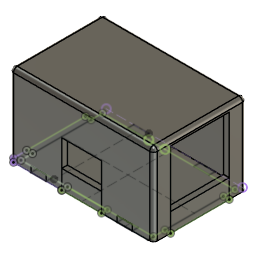
Thermux Temperature Node (Autodesk Fusion 360 design; units mm, degrees)
Autodesk Fusion 360 part; units mm, degrees
note: some values were not read from the file. Chosen so that the rebuilt part matches the saved one: which face or edge a step refers to.
sketch "Sketch1" plane through (0, 0, 0) normal (0, 0, 1) x (1, 0, 0) in component "Lid"
  line L0 (-19, 12.25) -> (19, 12.25)
  line L1 (19, 12.25) -> (19, -12.25)
  line L2 (19, -12.25) -> (-19, -12.25)
  line L3 (-19, -12.25) -> (-19, 12.25)
  line L4 (-19, 12.25) -> (19, -12.25) construction
  line L5 (19, 12.25) -> (-19, -12.25) construction
  line L6 (-17.5, 10.75) -> (17.5, 10.75)
  line L7 (17.5, 10.75) -> (17.5, -10.75)
  line L8 (17.5, -10.75) -> (-17.5, -10.75)
  line L9 (-17.5, -10.75) -> (-17.5, 10.75)
  line L10 (-5.25, -10.75) -> (5.25, -10.75)
  line L11 (5.25, -10.75) -> (5.25, -12.25)
  line L12 (5.25, -12.25) -> (-5.25, -12.25)
  line L13 (-5.25, -12.25) -> (-5.25, -10.75)
  line L14 (0, 12.25) -> (0, -12.25) construction
  line L15 (-19, 0) -> (19, 0) construction
  line L16 (-19, 7.75) -> (-17.5, 7.75)
  line L17 (-17.5, 7.75) -> (-17.5, -7.75)
  line L18 (-17.5, -7.75) -> (-19, -7.75)
  line L19 (-19, -7.75) -> (-19, 7.75)
  line L20 (17.5, 7.75) -> (19, 7.75)
  line L21 (19, 7.75) -> (19, -7.75)
  line L22 (19, -7.75) -> (17.5, -7.75)
  line L23 (17.5, -7.75) -> (17.5, 7.75)
  circle A0 centre (-3.125, 8.125) radius 1.125
  circle A1 centre (-3.125, 8.125) radius 2.125
  line L24 (-4.25, 12.25) -> (-4.25, -12.25) construction
  line L25 (-17.5, 9.25) -> (17.5, 9.25) construction
  line L26 (-5.25, 8.125) -> (-5.25, 10.75)
  line L27 (-1, 8.125) -> (-1, 10.75)
  dimension "d3" = 1.5
  dimension "d4" = 10.5
  dimension "d7" = 15.5
  dimension "d8" = 15.5
  dimension "d9" = 2.25
  dimension "d10" = 1
  dimension "d11" = 13.25
  dimension "d12" = 1.5
  dimension "d34" = 35
  dimension "d35" = 21.5
  constraint horizontal L0
  constraint perpendicular L0 L1
  constraint parallel L0 L2
  constraint parallel L1 L3
  constraint coincident L4 origin
  constraint coincident L5 origin
  constraint horizontal L10
  constraint vertical L11
  constraint horizontal L12
  constraint vertical L13
  constraint coincident L2 L11.end
  constraint coincident L8 L10.start
  constraint midpoint L0 L14.start
  constraint midpoint L2 L14.end
  constraint symmetric L11 L13 L14
  constraint midpoint L3 L15.start
  constraint midpoint L1 L15.end
  constraint horizontal L16
  constraint vertical L17
  constraint horizontal L18
  constraint vertical L19
  constraint coincident L9 L17.end
  constraint coincident L3 L16.start
  constraint horizontal L20
  constraint vertical L21
  constraint horizontal L22
  constraint vertical L23
  constraint coincident L1 L21.end
  constraint coincident L7 L20.start
  constraint symmetric L15 L16 L18
  constraint symmetric L15 L20 L22
  constraint coincident L0 L24.start
  constraint coincident L2 L24.end
  constraint perpendicular L2 L24
  constraint coincident L9 L25.start
  constraint coincident L7 L25.end
  constraint perpendicular L7 L25
  constraint tangent A0 L25
  constraint tangent A0 L24
  constraint coincident L6 L26.end
  constraint perpendicular L6 L26
  constraint coincident L6 L27.end
  constraint perpendicular L6 L27
  constraint coincident A1 L27.start
  constraint tangent A1 L27
  constraint tangent A1 L26
  constraint coincident A1 L26.start
  measures "d4" distance of L11 L13
  measures "d7" distance of L16 L18
  measures "d8" distance of L20 L22
  measures "d9" diameter of A0
  measures "d11" distance of L17 L24
  measures "d12" distance of L6 L25
  measures "d34" distance of L7 L9
  measures "d35" distance of L6 L8
extrude "Extrude4" add sketch "Sketch1" along normal blind 1.5 contours L0 L1 L3 L6 L7 L9 L16 L20 | L3 L9 L16 L17 L18 L19 | L1 L7 L20 L21 L22 L23 | L2 L3 L8 L9 L13 L18 | L6 L7 L8 L9 L10 L17 L23 A1 L26 L27 | L1 L2 L7 L8 L11 L22 | L2 L8 L10 L11 L12 L13 | L6 A1 L26 L27 | A1 | A0 makes body 1 in component "Lid"
extrude "Extrude5" add sketch "Sketch1" against normal blind 20 contours L0 L1 L3 L6 L7 L9 L16 L20 | L2 L3 L8 L9 L13 L18 | L1 L2 L7 L8 L11 L22 bodies 1 in component "Lid"
extrude "Extrude7" add sketch "Sketch1" against normal blind 8 contours L2 L8 L10 L11 L12 L13 bodies 1 in component "Lid"
fillet "Fillet1" radius 1 8 edges at (-19, -12.25, -9.25) (-19, 0, 1.5) (-19, 12.25, -9.25) (19, -12.25, -9.25) (19, 12.25, -9.25) (19, 0, 1.5) (0, -12.25, 1.5) (0, 12.25, 1.5) on bodies 1 in component "Lid"
sketch "Sketch1 (2)" plane through (0, 0, -20) normal (0, 0, 1) x (1, 0, 0) in component "Base"
  line L0 (5.25, -12.25) -> (-5.25, -12.25)
  line L1 (-5.25, -12.25) -> (-5.25, -10.75)
  line L2 (-5.25, -10.75) -> (5.25, -10.75)
  line L3 (5.25, -10.75) -> (5.25, -12.25)
  line L4 (-5.25, 10.75) -> (-1, 10.75)
  line L5 (-1, 10.75) -> (17.5, 10.75)
  line L6 (17.5, 10.75) -> (17.5, 7.75)
  line L7 (17.5, 7.75) -> (19, 7.75)
  line L8 (19, 7.75) -> (19, -7.75)
  line L9 (19, -7.75) -> (17.5, -7.75)
  line L10 (17.5, -7.75) -> (17.5, -10.75)
  line L11 (17.5, -10.75) -> (-17.5, -10.75)
  line L12 (-17.5, -10.75) -> (-17.5, -7.75)
  line L13 (-17.5, -7.75) -> (-19, -7.75)
  line L14 (-19, -7.75) -> (-19, 7.75)
  line L15 (-19, 7.75) -> (-17.5, 7.75)
  line L16 (-17.5, 7.75) -> (-17.5, 10.75)
  line L17 (-17.5, 10.75) -> (-5.25, 10.75)
  line L18 (-17.5, -7.75) -> (-17.5, 7.75)
  line L19 (17.5, -7.75) -> (17.5, 7.75)
  arc A0 (-19, -11.25) -> (-18, -12.25) centre (-18, -11.25) ccw
  line L20 (-19, -11.25) -> (-19, -7.75)
  line L21 (-19, -7.75) -> (-17.5, -7.75)
  line L22 (-17.5, -7.75) -> (-17.5, -10.75)
  line L23 (-17.5, -10.75) -> (-5.25, -10.75)
  line L24 (-5.25, -10.75) -> (-5.25, -12.25)
  line L25 (-5.25, -12.25) -> (-18, -12.25)
  line L26 (18, 12.25) -> (-18, 12.25) construction
  line L27 (0, -12.25) -> (0, 12.25) construction
  line L28 (-10.75, 10.75) -> (-6.75, 10.75)
  line L29 (-6.75, 10.75) -> (-6.75, 12.25)
  line L30 (-6.75, 12.25) -> (-10.75, 12.25)
  line L31 (-10.75, 12.25) -> (-10.75, 10.75)
  line L32 (-8.75, 10.75) -> (-8.75, -10.75) construction
  line L33 (10.75, 10.75) -> (6.75, 10.75)
  line L34 (6.75, 10.75) -> (6.75, 12.25)
  line L35 (10.75, 12.25) -> (10.75, 10.75)
  line L36 (6.75, 12.25) -> (10.75, 12.25)
  line L37 (-17.5, 0) -> (17.5, 0) construction
  line L38 (17.5, -10.75) -> (17.5, -12.25)
  line L39 (17.5, -12.25) -> (5.25, -12.25)
  line L40 (11.375, -12.25) -> (11.375, -10.75) construction
  line L41 (13.375, -10.75) -> (9.375, -10.75)
  line L42 (9.375, -10.75) -> (9.375, -12.25)
  line L43 (9.375, -12.25) -> (13.375, -12.25)
  line L44 (13.375, -12.25) -> (13.375, -10.75)
  line L45 (-13.375, -12.25) -> (-13.375, -10.75)
  line L46 (-13.375, -10.75) -> (-9.375, -10.75)
  line L47 (-9.375, -12.25) -> (-13.375, -12.25)
  line L48 (-9.375, -10.75) -> (-9.375, -12.25)
  dimension "d63" = 4
  constraint coincident L12.end L13.start
  constraint coincident L15.end L16.start
  constraint coincident L9.end L10.start
  constraint coincident L6.end L7.start
  constraint midpoint L0 L27.start
  constraint midpoint L26 L27.end
  constraint horizontal L28
  constraint vertical L29
  constraint horizontal L30
  constraint vertical L31
  constraint coincident L26 L29.end
  constraint coincident L17 L28.start
  constraint coincident L17 L32.start
  constraint coincident L23 L32.end
  constraint perpendicular L23 L32
  constraint symmetric L27 L28.start L33.start
  constraint symmetric L27 L28.end L33.end
  constraint symmetric L27 L29.end L34.end
  constraint symmetric L27 L30.end L35.start
  constraint midpoint L18 L37.start
  constraint midpoint L19 L37.end
  constraint coincident L10.end L11.start
  constraint perpendicular L0 L38
  constraint coincident L0.start L3.end
  constraint perpendicular L38 L39
  constraint midpoint L39 L40.start
  constraint coincident L11 L40.end
  constraint perpendicular L11 L40
  constraint horizontal L41
  constraint vertical L42
  constraint horizontal L43
  constraint vertical L44
  constraint coincident L39 L42.end
  constraint coincident L11 L41.start
  constraint equal L36 L43
  constraint symmetric L40 L42 L44
  constraint symmetric L27 L41.start L45.end
  constraint symmetric L27 L41.end L46.end
  constraint symmetric L27 L42.end L47.start
  constraint symmetric L27 L43.end L45.start
  measures "d63" distance of L29.end L30.end
extrude "Extrude1" add sketch "Sketch1 (2)" along normal blind 5 separate body contours L0 L1 L2 L3 L11 L24 | L7 L8 L9 L19 | L13 L14 L15 L18 L21 makes body 2 at (-17.5, -2.5833, -18.3333) makes body 3 at (17.5, -2.5833, -18.3333) makes body 4 at (1.75, -12.25, -18.3333) in component "Base"
extrude "Extrude2" add sketch "Sketch1 (2)" along normal blind 1.5 contours L2 L4 L5 L6 L10 L11 L12 L16 L17 L18 L19 L22 L23 L28 L33 L41 L46 bodies 2 3 4 in component "Base"
extrude "Extrude9" add sketch "Sketch1 (2)" along normal up to surface (1.5 mm away) contours L2 L4 L5 L6 L10 L11 L12 L16 L17 L18 L19 L22 L23 L28 L33 L41 L46 | L11 L39 L41 L42 L43 L44 | L11 L23 L25 L45 L46 L47 L48 | L5 L33 L34 L35 L36 | L17 L28 L29 L30 L31 bodies 2 in component "Base"
extrude "Extrude9'" cut sketch "Sketch1 (2)" along normal up to surface (1.5 mm away) contours L11 L39 L41 L42 L43 L44 | L11 L23 L25 L45 L46 L47 L48 | L5 L33 L34 L35 L36 | L17 L28 L29 L30 L31 bodies 1 in component "Lid"
component "Lid" placed x (1, 0, 0) y (0, 1, 0) z (0, 0, 1) at (0, 0, 0)
component "Base" placed x (1, 0, 0) y (0, 1, 0) z (0, 0, 1) at (0, 0, 0)
